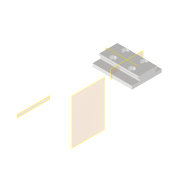
# Autodesk Inventor part: 40_Cube_Z-only_illuminationarm_base-wifiholder_slidermount
Saved by Autodesk Inventor 2022 (Build 260153000, 153)
## iProperties
Created: 2022-12-09
Part Number: 40_Cube_Z-only_illuminationarm_base-wifiholder_slidermount
Material: Generisch
Document SubType Name: Modeling
Designer: diederichbenedict
Density: 1 g/cm^3
Appearance: Vorgabe
Author: diederichbenedict
Autodesk Inventor part; units mm, degrees
ref_plane "YZ Plane" through (0, 0, 0) normal (1, 0, 0) x (0, 1, 0)
ref_plane "XZ Plane" through (0, 0, 0) normal (0, 1, 0) x (-1, 0, 0)
ref_plane "XY Plane" through (0, 0, 0) normal (0, 0, 1) x (1, 0, 0)
ref_plane "Arbeitsebene9" through (-58.9003, 150.915, -19.5294) normal (1, 0, 0) x (0, 1, 0.0002861)
ref_plane "Arbeitsebene10" through (-3.3213, 95.2, -15) normal (1, 0, 0) x (0, 1, 0)
sketch "Skizze8" plane through (-3.3213, 95.2, -15) normal (1, 0, 0) x (0, 1, 0)
  line L0 (51.0327, -12.5388) -> (54.3913, -9.7235)
  line L1 (55.2125, -10.1069) -> (55.2018, -30.9624)
  line L2 (54.3802, -31.345) -> (51.0244, -28.5262)
  line L3 (50.2028, -28.9088) -> (50.1999, -34.5321)
  line L4 (50.2154, -4.5321) -> (50.2115, -12.1553)
  line L5 (50.2154, -13.2238) -> (55.2125, -9.0351)
  line L6 (55.2125, -9.0351) -> (55.2125, -32.0442)
  line L7 (55.2125, -32.0442) -> (50.2154, -27.8467)
  line L8 (50.2154, -13.2238) -> (50.2154, -27.8467)
  line L9 (54.9125, -9.678) -> (50.5154, -13.3638)
  line L10 (50.5154, -13.3638) -> (50.5154, -27.7069)
  line L11 (50.5154, -27.7069) -> (54.9125, -31.4004)
  line L12 (54.9125, -31.4004) -> (54.9125, -9.678)
  line L13 (50.5154, -13.3638) -> (46.5154, -13.3638)
  line L14 (50.5154, -13.3638) -> (54.5154, -13.3638) construction
  line L15 (46.5154, -13.3638) -> (46.5154, -27.7069)
  line L16 (46.5154, -27.7069) -> (50.5154, -27.7069)
  line L17 (67.5498, -4.541) -> (50.2154, -4.5321)
  line L18 (61.046, -34.5285) -> (50.2065, -34.5303)
  line L19 (46.5154, -13.3638) -> (49.8154, -13.3638)
  line L20 (49.8154, -13.3638) -> (49.8154, -4.5318)
  line L21 (49.8154, -4.5318) -> (46.5154, -4.5318)
  line L22 (46.5154, -4.5318) -> (46.5154, -13.3638)
  line L23 (46.5154, -27.7069) -> (49.8154, -27.7069)
  line L24 (49.8154, -27.7069) -> (49.8154, -34.5304)
  line L25 (49.8154, -34.5304) -> (46.5154, -34.5304)
  line L26 (46.5154, -34.5304) -> (46.5154, -27.7069)
  point P0 (-95.2, 15)
  point P1 (50.2154, -27.7069)
  point P2 (54.3913, -9.7235)
  point P3 (50.2154, -13.3638)
  dimension "d62" = 0.3
  dimension "d63" = 4
  dimension "d64" = 180
  dimension "d65" = 0.4
  constraints: 54 end point, 4 horizontal, 4 parallel, 4 perpendicular, 2 vertical, 1 collinear, 1 point on line, 23 other
  measures "d62" distance between parallel lines of L5 L9
  measures "d63" distance of L9.end L13.end
  measures "d64" angle of L14 L13
  measures "d65" distance from line of L7.end L24
extrude "Extrusion5" add sketch "Skizze8" along normal blind 40 contours L13 L10 L16 L8 | L8 L16 L15 L13 | L9 L12 L11 L10 | L13 L22 L21 L20 | L24 L25 L26 L16
sketch "Skizze9" plane through (-3.3213, 150.1125, -5.7071) normal (0, 1, 0) x (1, 0, 0)
  line L0 (10.4, 23.7321) -> (29.6, 23.7321)
  line L1 (29.6, 23.7321) -> (29.6, 35.9321)
  line L2 (29.6, 35.9321) -> (10.4, 35.9321)
  line L3 (10.4, 35.9321) -> (10.4, 23.7321)
  line L4 (10.4, 23.7321) -> (29.6, 35.9321) construction
  line L5 (29.6, 23.7321) -> (10.4, 35.9321) construction
  line L6 (0, 40.6933) -> (0, 18.9709) projected
  line L7 (0, 18.9709) -> (40, 18.9709) projected
  line L8 (40, 40.6933) -> (40, 18.9709) projected
  line L9 (0, 40.6933) -> (40, 40.6933) projected
  point P0 (3.3213, -5.7071)
  point P1 (20, 29.8321)
  dimension "d52" = 19.2
  dimension "d53" = 12.2
  constraints: 12 end point, 4 coincident, 2 midpoint, 2 parallel, 1 horizontal, 1 perpendicular
  measures "d52" distance of L2.end L1.end
  measures "d53" distance of L1.end L0.end
fillet "Rundung3" radius 1 5 edges at (16.6787, 150.1125, -24.678) (16.6787, 150.1125, -46.4004) (16.6787, 145.0154, -42.7069) (16.6787, 145.7154, -28.3638) (16.6787, 145.0154, -28.3638)
hole "Bohrung4" at (7.0787, 150.1125, -29.4392) at (26.2787, 150.1125, -29.4392) at (26.2787, 150.1125, -41.6392) at (7.0787, 150.1125, -41.6392) direction (0, -1, 0) diameter 2.8 end through all counterbore diameter 6 counterbore depth 3.53
ref_plane "Arbeitsebene11" through (-3.3213, 141.7154, -34.5311) normal (0, 0, 1) x (1, 0, 0)
ref_plane "Arbeitsebene12" through (16.6787, 95.2, -15) normal (1, 0, 0) x (0, 0, -1)
